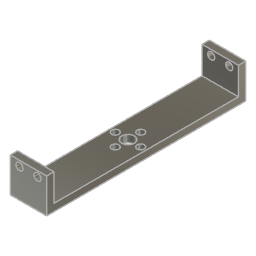
nerfaccelp2 v1 (Autodesk Fusion 360 design; units mm, degrees)
Autodesk Fusion 360 part; units mm, degrees
note: some values were not read from the file. Set by a fixed rule: which sketch regions a step uses.
sketch "Sketch1" plane through (0, 0, 0) normal (1, 0, 0) x (0, 1, 0)
  line L0 (-50.7, 0) -> (50.7, 0)
  line L1 (-50.7, 0) -> (-50.7, 15)
  line L2 (-50.7, 15) -> (-54.7, 15)
  line L3 (-54.7, 15) -> (-54.7, -4)
  line L4 (-54.7, -4) -> (54.7, -4)
  line L5 (54.7, -4) -> (54.7, 15)
  line L6 (54.7, 15) -> (50.7, 15)
  line L7 (50.7, 15) -> (50.7, 0)
  dimension "d1" = 101.4
  dimension "d2" = 15
  dimension "d3" = 4
  dimension "d4" = 4
  dimension "d5" = 4
  constraint horizontal L0
  constraint midpoint origin L0
  constraint vertical L1
  constraint perpendicular L1 L2
  constraint perpendicular L2 L3
  constraint perpendicular L3 L4
  constraint perpendicular L4 L5
  constraint perpendicular L5 L6
  constraint vertical L7
  constraint equal L1 L7
  measures "d1" distance of L0.start L0.end
  measures "d2" distance of L0.start L1.end
  measures "d3" distance of L1.end L2.end
  measures "d4" distance of L5.end L6.end
  measures "d5" vertical distance of L0.start L3.end
extrude "Extrude1" add sketch "Sketch1" along normal blind 20
sketch "Sketch2" plane through (0, -54.7, 0) normal (0, -1, 0) x (1, 0, 0)
  line L0 (0, 15) -> (0, -4)
  line L1 (0, -4) -> (20, -4)
  line L2 (20, -4) -> (20, 15)
  line L3 (20, 15) -> (0, 15)
  line L4 (7, 12.05) -> (13, 12.05)
  line L5 (3.1, 12.05) -> (16.9, 12.05)
  circle A0 centre (5.05, 12.05) radius 1.95
  circle A1 centre (14.95, 12.05) radius 1.95
  line L6 (10, 12.05) -> (10, 15)
  line L7 (5.05, 14) -> (10, 14)
  dimension "d8" = 6
  dimension "d9" = 13.8
  dimension "d10" = 1
  constraint perpendicular L0 L4
  constraint midpoint L4 L5
  constraint horizontal L5
  constraint coincident L5 A0.centre
  constraint coincident L4.start A0
  constraint coincident L5.start A0
  constraint coincident L5 A1.centre
  constraint coincident L5.end A1
  constraint coincident L4.end A1
  constraint midpoint L5 L6.start
  constraint midpoint L3 L6.end
  constraint vertical L6
  constraint coincident A0 L7.start
  constraint tangent A0 L7
  constraint coincident L6 L7.end
  constraint horizontal L7
  measures "d8" distance of L4.start L4.end
  measures "d9" distance of L5.start L5.end
  measures "d10" distance of L6.end L7.end
extrude "Extrude2" cut sketch "Sketch2" against normal blind 109.4 contours L5 A0 | L5 A0 | L5 A1 | L5 A1
sketch "Sketch3" plane through (0, 0, 0) normal (0, 0, 1) x (-1, 0, 0)
  line L0 (0, -50.7) -> (0, 50.7)
  line L1 (0, 50.7) -> (-20, 50.7)
  line L2 (-20, 50.7) -> (-20, -50.7)
  line L3 (-20, -50.7) -> (0, -50.7)
  line L4 (0, 0) -> (-20, 0)
  line L5 (-10, 0) -> (-10, -5.6)
  line L6 (-10, 0) -> (-10, -8.4)
  circle A0 centre (-10, -7) radius 1.4
  circle A1 centre (-10, -7) radius 2
  circle A2 centre (-3, 0) radius 2
  circle A3 centre (-10, 7) radius 2
  circle A4 centre (-17, 0) radius 2
  circle A5 centre (-10, 0) radius 3.5
  dimension "d13" = 5.6
  dimension "d14" = 8.4
  dimension "d15" = 4
  dimension "d17" = 360
  dimension "d20" = 7
  constraint midpoint L2 L4.end
  constraint perpendicular L2 L4
  constraint midpoint L4 L5.start
  constraint perpendicular L4 L5
  constraint perpendicular L4 L6
  constraint coincident L6 A0.centre
  constraint coincident L5.end A0
  constraint coincident L6.end A0
  constraint coincident L4.start origin
  constraint concentric A0 A1
  constraint coincident L5.start L6.start
  measures "d13" distance of L5.start L5.end
  measures "d14" distance of L5.start L6.end
  measures "d15" diameter of A1
  measures "d20" diameter of A5
extrude "Extrude3" cut sketch "Sketch3" against normal blind 4 contours L4 A2 | L4 A2 | L4 A4 | L4 A4 | L4 L5 L6 A5 | L4 A5 | L4 L5 L6 A5 | L6 A0 | L6 A0 | A1 | A3
equation "d13 = ( 11.2 / 2 ) * 1 mm"
equation "d14 = ( 16.8 / 2 ) * 1 mm"
